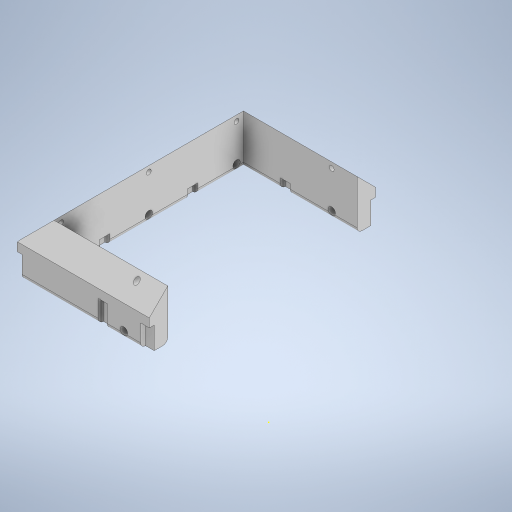
# Autodesk Inventor part: Palm_FingerAttachment
Saved by Autodesk Inventor 2023 (Build 270158000, 158)
## iProperties
Created: 2023-04-19
Part Number: Palm_FingerAttachment
Material: Generic
Document SubType Name: Modeling
Designer: 1senadi
Density: 1 g/cm^3
Appearance: Default
Author: 1senadi
Autodesk Inventor part; units mm, degrees
ref_plane "YZ Plane" through (0, 0, 0) normal (1, 0, 0) x (0, 1, 0)
ref_plane "XZ Plane" through (0, 0, 0) normal (0, 1, 0) x (-1, 0, 0)
ref_plane "XY Plane" through (0, 0, 0) normal (0, 0, 1) x (1, 0, 0)
sketch "Sketch1" plane through (0, 0, 0) normal (0, 1, 0) x (-1, 0, 0)
  line L0 (0, 0) -> (102, 0)
  line L1 (102, 0) -> (102, 91.8)
  line L2 (102, 91.8) -> (0, 91.8)
  line L3 (0, 91.8) -> (0, 0)
  line L4 (94.5, 84.3) -> (94.5, 7.5)
  line L5 (94.5, 7.5) -> (7.5, 7.5)
  line L6 (7.5, 7.5) -> (7.5, 84.3)
  line L7 (7.5, 84.3) -> (94.5, 84.3)
  dimension "d0" = 102
  dimension "d1" = 91.8
  dimension "d2" = 7.5
  constraints: 16 end point, 4 parallel, 2 perpendicular, 1 horizontal, 3 other
  measures "d0" distance of L2.end L1.end
  measures "d1" distance of L1.end L0.end
  measures "d2" distance between parallel lines of L1 L4
extrude "Extrusion1" add sketch "Sketch1" along normal blind 20
sketch "Sketch2" plane through (-102, 0, 0) normal (-1, 0, 0) x (0, 0, 1)
  line L0 (0, 0) -> (0, 9)
  line L1 (0, 0) -> (0, 20) projected
  line L2 (0, 9) -> (3.5, 9)
  line L3 (3.5, 9) -> (3.5, 0)
  line L4 (91.8, 0) -> (0, 0) projected
  line L5 (0, 0) -> (3.5, 0)
  line L6 (3.5, 0) -> (17.1, 0)
  line L7 (17.1, 0) -> (17.1, 9)
  line L8 (17.1, 9) -> (20.6, 9)
  line L9 (20.6, 9) -> (20.6, 0)
  line L10 (17.1, 0) -> (20.6, 0)
  line L11 (56.2, 9) -> (56.2, 0)
  line L12 (52.7, 9) -> (56.2, 9)
  line L13 (52.7, 0) -> (52.7, 9)
  line L14 (52.7, 0) -> (56.2, 0)
  line L15 (39.1, 0) -> (52.7, 0)
  line L16 (39.1, 9) -> (39.1, 0)
  line L17 (35.6, 9) -> (39.1, 9)
  line L18 (35.6, 0) -> (35.6, 9)
  line L19 (35.6, 0) -> (39.1, 0)
  line L20 (91.8, 9) -> (91.8, 0)
  line L21 (88.3, 9) -> (91.8, 9)
  line L22 (88.3, 0) -> (88.3, 9)
  line L23 (88.3, 0) -> (91.8, 0)
  line L24 (74.7, 0) -> (88.3, 0)
  line L25 (74.7, 9) -> (74.7, 0)
  line L26 (71.2, 9) -> (74.7, 9)
  line L27 (71.2, 0) -> (71.2, 9)
  line L28 (71.2, 0) -> (74.7, 0)
  point P0 (88.3, 0)
  point P1 (74.7, 0)
  point P2 (52.7, 0)
  point P3 (39.1, 0)
  dimension "d5" = 9
  dimension "d6" = 3.5
  dimension "d7" = 13.6
  dimension "d8" = 9
  dimension "d9" = 3.5
  dimension "d12" = 35.6
  constraints: 54 end point, 6 perpendicular, 4 point on line, 1 collinear, 1 horizontal, 34 other
  measures "d5" distance of L0.start L0.end
  measures "d6" distance of L0.end L2.end
  measures "d7" distance of L3.end L6.end
  measures "d8" distance of L6.end L7.end
  measures "d9" distance of L7.end L8.end
  measures "d12" distance of L8.end L11.start
extrude "Extrusion2" cut sketch "Sketch2" against normal blind 2
sketch "Sketch3" plane through (-102, 20, 91.8) normal (0, 0, 1) x (1, 0, 0)
  point P0 (102, -20)
sketch "Sketch4" plane through (-102, 20, 91.8) normal (0, 0, 1) x (1, 0, 0)
  line L0 (2, -20) -> (0, -20) projected
  line L1 (2, -20) -> (33.013, -20)
  line L2 (7.5, -20) -> (94.5, -20) projected
  line L3 (33.013, -20) -> (33.013, -11)
  line L4 (33.013, -11) -> (36.513, -11)
  line L5 (36.513, -11) -> (36.513, -20)
  line L6 (33.013, -20) -> (36.513, -20)
  line L7 (36.513, -20) -> (50.113, -20)
  line L8 (50.113, -20) -> (50.113, -11)
  line L9 (50.113, -11) -> (53.613, -11)
  line L10 (53.613, -11) -> (53.613, -20)
  line L11 (53.613, -20) -> (50.113, -20)
  point P0 (102, -20)
  dimension "d19" = 31.013
  dimension "d20" = 9
  dimension "d21" = 3.5
  dimension "d22" = 13.6
  dimension "d23" = 9
  dimension "d24" = 3.5
  constraints: 20 end point, 6 point on line, 3 perpendicular, 2 collinear, 1 vertical
  measures "d19" distance of L0.start L1.end
  measures "d20" distance of L1.end L3.end
  measures "d21" distance of L3.end L4.end
  measures "d22" distance of L5.end L7.end
  measures "d23" distance of L7.end L8.end
  measures "d24" distance of L8.end L9.end
extrude "Extrusion3" cut sketch "Sketch4" against normal blind 2
ref_plane "Work Plane1" through (-102, 0, 45.9) normal (0, 0, 1) x (1, 0, 0)
sketch "Sketch5" plane through (0, 0, 0) normal (0, -1, 0) x (1, 0, 0)
  line L0 (0, 0) -> (-100, 0) projected
  line L1 (0, 91.8) -> (0, 0) projected
  line L2 (-48.387, 91.8) -> (0, 91.8) projected
  line L3 (-48.387, 91.8) -> (-48.387, 89.8) projected
  line L4 (-48.387, 89.8) -> (-51.887, 89.8) projected
  line L5 (-51.887, 89.8) -> (-51.887, 91.8) projected
  line L6 (-65.487, 91.8) -> (-51.887, 91.8) projected
  line L7 (-65.487, 91.8) -> (-65.487, 89.8) projected
  line L8 (-65.487, 89.8) -> (-68.987, 89.8) projected
  line L9 (-68.987, 89.8) -> (-68.987, 91.8) projected
  line L10 (-100, 91.8) -> (-68.987, 91.8) projected
  line L11 (-100, 91.8) -> (-100, 88.3) projected
  line L12 (-100, 88.3) -> (-102, 88.3) projected
  line L13 (-102, 74.7) -> (-102, 88.3) projected
  line L14 (-102, 74.7) -> (-100, 74.7) projected
  line L15 (-100, 74.7) -> (-100, 71.2) projected
  line L16 (-100, 71.2) -> (-102, 71.2) projected
  line L17 (-102, 56.2) -> (-102, 71.2) projected
  line L18 (-102, 56.2) -> (-100, 56.2) projected
  line L19 (-100, 56.2) -> (-100, 52.7) projected
  line L20 (-100, 52.7) -> (-102, 52.7) projected
  line L21 (-102, 39.1) -> (-102, 52.7) projected
  line L22 (-102, 39.1) -> (-100, 39.1) projected
  line L23 (-100, 39.1) -> (-100, 35.6) projected
  line L24 (-100, 35.6) -> (-102, 35.6) projected
  line L25 (-102, 20.6) -> (-102, 35.6) projected
  line L26 (-102, 20.6) -> (-100, 20.6) projected
  line L27 (-100, 20.6) -> (-100, 17.1) projected
  line L28 (-100, 17.1) -> (-102, 17.1) projected
  line L29 (-102, 3.5) -> (-102, 17.1) projected
  line L30 (-102, 3.5) -> (-100, 3.5) projected
  line L31 (-100, 3.5) -> (-100, 0) projected
  line L32 (-94.5, 84.3) -> (-94.5, 7.5) projected
  line L33 (-7.5, 84.3) -> (-94.5, 84.3) projected
  line L34 (-7.5, 7.5) -> (-7.5, 84.3) projected
  line L35 (-94.5, 7.5) -> (-7.5, 7.5) projected
  line L36 (-59.4, 0) -> (-59.4, 2) projected
  line L37 (-48.387, 91.8) -> (-48.387, 89.8) projected
  line L38 (-102, 91.8) -> (0, 91.8) projected
  line L39 (-48.387, 91.8) -> (0, 91.8)
  line L40 (0, 91.8) -> (0, 0)
  line L41 (-48.387, 0) -> (0, 0)
  line L42 (-48.387, 91.8) -> (-48.387, 0)
  line L43 (0, 0) -> (-102, 0) projected
  line L44 (-48.387, 0) -> (0, 0)
  point P0 (-80, 0)
  point P1 (-76.5, 0)
  point P2 (-62.9, 0)
  constraints: 10 end point, 2 collinear, 2 perpendicular, 2 other
extrude "Extrusion4" cut sketch "Sketch5" against normal up to surface (20 mm away) contours L0 L42 L35 L34 L33 L3 L2 L1 | L42 L33 L34 L35
sketch "Sketch6" plane through (-102, 9, 91.8) normal (0, 0, 1) x (1, 0, 0)
  line L0 (0, 11) -> (53.613, 11) projected
  line L1 (0, 11) -> (0, 3.5)
  line L2 (0, 0) -> (0, 11) projected
  line L3 (0, 3.5) -> (7.5, 11)
  line L4 (7.5, 11) -> (0, 11)
  point P0 (102, -9)
  point P1 (42.6, 11)
  point P2 (7.5, 11)
  point P3 (2, 11)
  dimension "d29" = 7.5
  dimension "d30" = 45
  constraints: 6 end point, 1 perpendicular, 1 point on line
  measures "d29" distance of L0.start L1.end
  measures "d30" angle of L3 L1
extrude "Extrusion5" cut sketch "Sketch6" against normal up to surface (91.8 mm away)
sketch "Sketch8" plane through (-102, 0, 20.6) normal (-1, 0, 0) x (0, 0, 1)
  line L0 (54.1, 0) -> (67.7, 0) projected
  line L1 (60.9, 0) -> (60.9, 2.75)
  line L2 (60.9, 0) -> (63.65, 0) construction
  circle A0 centre (60.9, 2.75) radius 1.5
  line L3 (60.9, 2.75) -> (60.9, 20)
  line L4 (-20.6, 20) -> (71.2, 20) projected
  line L5 (60.9, 20) -> (60.9, 17.75)
  circle A1 centre (60.9, 17.75) radius 1
  circle A2 centre (25.3, 2.75) radius 1.5
  circle A3 centre (25.3, 17.75) radius 1
  circle A4 centre (-10.3, 2.75) radius 1.5
  circle A5 centre (-10.3, 17.75) radius 1
  point P0 (-20.6, 0)
  point P1 (-13.1, 20)
  point P2 (63.7, 20)
  dimension "d38" = 2.75
  dimension "d39" = 90
  dimension "d40" = 3
  dimension "d41" = 2.25
  dimension "d42" = 2
  dimension "d45" = 35.6
  constraints: 8 end point, 6 centre point, 2 coincident, 2 horizontal, 2 point on line, 2 vertical, 1 midpoint, 1 perpendicular, 8 other
  measures "d38" distance of L1.start L1.end
  measures "d39" angle of L2 L1
  measures "d40" diameter of A0
  measures "d41" distance of L3.end L5.end
  measures "d42" diameter of A1
  measures "d45" distance of L3.start A2.centre
extrude "Extrusion7" cut sketch "Sketch8" against normal up to surface (7.5 mm away)
sketch "Sketch9" plane through (-102, 9, 91.8) normal (0, 0, 1) x (1, 0, 0)
  line L0 (36.513, -9) -> (50.113, -9) projected
  line L1 (43.313, -9) -> (43.313, -6.25)
  circle A0 centre (43.313, -6.25) radius 1.5
  line L2 (7.5, 11) -> (42.6, 11) projected
  line L3 (43.313, -9) -> (43.313, 11)
  line L4 (7.5, 11) -> (53.613, 11) projected
  line L5 (43.313, 11) -> (43.313, 8.75)
  circle A1 centre (43.313, 8.75) radius 1
  point P0 (102, -9)
  point P1 (43.4998, 11)
  dimension "d52" = 2.75
  dimension "d53" = 3
  dimension "d54" = 2.25
  dimension "d55" = 2
  constraints: 6 end point, 2 centre point, 2 coincident, 2 point on line, 1 midpoint, 1 perpendicular, 1 vertical
  measures "d52" distance of L1.start L1.end
  measures "d53" diameter of A0
  measures "d54" distance of L3.end L5.end
  measures "d55" diameter of A1
extrude "Extrusion8" cut sketch "Sketch9" against normal up to surface (7.5 mm away)
mirror "Mirror2" about plane through (-102, 0, 45.9) normal (0, 0, 1) of "Extrusion8", "Extrusion3"
sketch "Sketch12" plane through (0, 0, 0) normal (0, -1, 0) x (1, 0, 0)
  line L0 (-100, 20.6) -> (-100, 17.1) projected
  line L1 (-100, 39.1) -> (-100, 35.6) projected
  line L2 (-100, 20.6) -> (-100, 35.6)
  line L3 (-100, 35.6) -> (-94.5, 35.6)
  line L4 (-94.5, 84.3) -> (-94.5, 7.5) projected
  line L5 (-100, 28.1) -> (-94.5, 28.1)
  line L6 (-94.5, 28.1) -> (-94.5, 26.1)
  line L7 (-94.5, 28.1) -> (-94.5, 30.1)
  line L8 (-94.5, 30.1) -> (-96.5, 30.1)
  line L9 (-96.5, 30.1) -> (-96.5, 26.1)
  line L10 (-96.5, 26.1) -> (-94.5, 26.1)
  line L11 (-96.5, 61.7) -> (-94.5, 61.7)
  line L12 (-94.5, 63.7) -> (-94.5, 61.7)
  line L13 (-94.5, 63.7) -> (-94.5, 65.7)
  line L14 (-94.5, 65.7) -> (-96.5, 65.7)
  line L15 (-96.5, 65.7) -> (-96.5, 61.7)
  point P0 (0, 0)
  point P1 (-94.5, 8.6969)
  dimension "d71" = 2
  dimension "d72" = 2
  dimension "d73" = 2
  dimension "d76" = 35.6
  constraints: 26 end point, 4 perpendicular, 4 point on line, 2 vertical, 1 midpoint, 1 parallel, 10 other
  measures "d71" distance of L5.end L6.end
  measures "d72" distance of L5.end L7.end
  measures "d73" distance of L7.end L8.end
  measures "d76" distance of L9.end L11.start
extrude "Extrusion11" cut sketch "Sketch12" against normal blind 4 contours L9 L8 L4 L5 | L5 L4 L10 L9 | L4 L11 L15 L14
fillet "Fillet1" radius 2 5 edges at (-94.5, 0, 45.9) (-94.5, 0, 75) (-94.5, 0, 16.8) (-71.4435, 0, 7.5) (-71.4435, 0, 84.3)
fillet "Fillet2" radius 2 10 edges at (-58.687, 0, 0) (-84.4935, 0, 0) (-102, 0, 10.3) (-102, 0, 28.1) (-102, 0, 45.9) (-102, 0, 63.7) (-102, 0, 81.5) (-84.4935, 0, 91.8) (-58.687, 0, 91.8) (-102, 12.5, 45.9)
sketch "Sketch13" plane through (-48.387, 9, 91.8) normal (1, 0, 0) x (0, 0, -1)
  line L0 (7.5, 11) -> (15, 11) construction
  line L1 (0, 0) -> (0, 11) projected
  line L2 (0, 11) -> (0, 3.5)
  line L3 (0, 11) -> (7.5, 11) projected
  line L4 (0, 3.5) -> (7.5, 11)
  line L5 (7.5, 11) -> (0, 11)
  line L6 (7.5, 11) -> (84.3, 11) projected
  line L7 (45.9, 11) -> (45.9, -9)
  line L8 (91.8, 0) -> (91.8, 11)
  line L9 (91.8, 11) -> (84.3, 11)
  line L10 (91.8, 3.5) -> (84.3, 11)
  point P0 (91.8, -9)
  dimension "d88" = 7.5
  dimension "d89" = 45
  constraints: 16 end point, 3 point on line, 3 symmetric about line, 1 horizontal, 1 midpoint, 1 vertical
  measures "d88" distance of L1.end L2.end
  measures "d89" angle of L4 L2
extrude "Extrusion12" cut sketch "Sketch13" against normal up to surface (53.613 mm away)
sketch "Sketch15" plane through (0, 0, 0) normal (0, -1, 0) x (1, 0, 0)
  line L0 (-94.5, 84.3) -> (-94.5, 7.5) projected
  line L1 (-57.388, 84.3) -> (-48.387, 84.3) projected
  line L2 (-94.5, 84.3) -> (-48.387, 84.3)
  line L3 (-94.5, 84.3) -> (-59.986, 84.3) projected
  line L4 (-94.5, 84.3) -> (-79.5, 84.3)
  line L5 (-79.5, 84.3) -> (-79.5, 86.3)
  line L6 (-48.387, 86.3) -> (-96.5, 86.3) projected
  line L7 (-79.5, 86.3) -> (-75.5, 86.3)
  line L8 (-75.5, 86.3) -> (-75.5, 84.3)
  line L9 (-79.5, 84.3) -> (-75.5, 84.3)
  line L10 (-102, 52.7) -> (-102, 47.199) projected
  line L11 (-102, 44.601) -> (-102, 39.1) projected
  line L12 (-102, 0) -> (-102, 91.8) projected
  line L13 (-102, 45.9) -> (-44.6924, 45.9)
  line L14 (-102, 45.9) -> (-44.6924, 45.9) construction
  line L15 (-94.5, 7.5) -> (-48.387, 7.5)
  line L16 (-79.5, 7.5) -> (-79.5, 5.5)
  line L17 (-48.387, 5.5) -> (-96.5, 5.5)
  line L18 (-75.5, 5.5) -> (-75.5, 7.5)
  point P0 (0, 0)
  dimension "d92" = 15
  dimension "d93" = 4
  dimension "d94" = 0
  constraints: 24 end point, 7 symmetric about line, 4 point on line, 2 collinear, 2 horizontal, 2 perpendicular, 1 midpoint, 1 vertical, 1 vertical alignment
  measures "d92" distance of L0.start L4.end
  measures "d93" distance of L5.end L7.end
  measures "d94" distance between parallel lines of L13 L14
extrude "Extrusion13" cut sketch "Sketch15" against normal blind 4
body "Solid1"
